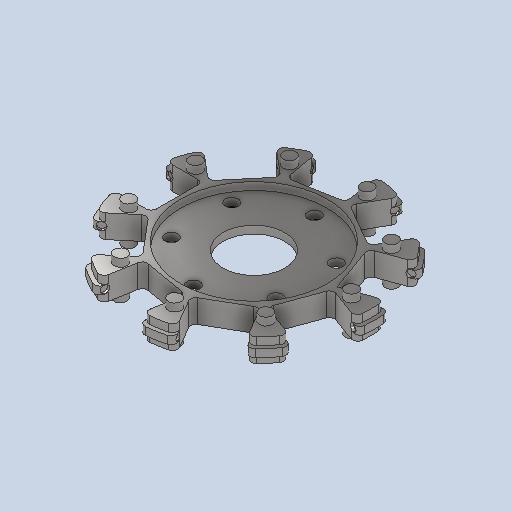
# Autodesk Inventor part: omuni_flame
Saved by Autodesk Inventor 2025.1 (Build 291241000, 241)
## iProperties
Created: 2023-11-21
Part Number: omuni_flame
Material: ステンレス鋼
Document SubType Name: Modeling
Designer: fhbdh
Density: 8 g/cm^3
Appearance: 半つや出し
Author: fhbdh
Autodesk Inventor part; units mm, degrees
ref_plane "YZ Plane" through (0, 0, 0) normal (1, 0, 0) x (0, 1, 0)
ref_plane "XZ Plane" through (0, 0, 0) normal (0, 1, 0) x (-1, 0, 0)
ref_plane "XY Plane" through (0, 0, 0) normal (0, 0, 1) x (1, 0, 0)
sketch "スケッチ1" plane through (0, 0, 0) normal (0, 1, 0) x (-1, 0, 0)
  circle A0 centre (0, 0) radius 12
  circle A1 centre (0, 0) radius 47
  line L0 (45.92385, 10) -> (29.92385, 10)
  line L1 (29.92385, 10) -> (29.92385, -10)
  line L2 (29.92385, -10) -> (45.92385, -10)
  line L3 (0, 0) -> (47, 0) construction
  line L4 (28.751834, 37.179726) -> (16.495123, 26.895124)
  line L5 (16.495123, 26.895124) -> (29.350875, 11.574236)
  line L6 (29.350875, 11.574236) -> (41.607586, 21.858837)
  line L7 (-1.873485, 46.962645) -> (-4.651856, 31.205721)
  line L8 (-4.651856, 31.205721) -> (15.0443, 27.732758)
  line L9 (15.0443, 27.732758) -> (17.82267, 43.489682)
  line L10 (-31.622179, 34.771221) -> (-23.622179, 20.914814)
  line L11 (-23.622179, 20.914814) -> (-6.301671, 30.914814)
  line L12 (-6.301671, 30.914814) -> (-14.301671, 44.771221)
  line L13 (-46.574504, 6.309956) -> (-31.539422, 0.837633)
  line L14 (-31.539422, 0.837633) -> (-24.69902, 19.631486)
  line L15 (-24.69902, 19.631486) -> (-39.734102, 25.103808)
  line L16 (-39.734102, -25.103808) -> (-24.69902, -19.631486)
  line L17 (-24.69902, -19.631486) -> (-31.539422, -0.837633)
  line L18 (-31.539422, -0.837633) -> (-46.574504, -6.309956)
  line L19 (-14.301671, -44.771221) -> (-6.301671, -30.914814)
  line L20 (-6.301671, -30.914814) -> (-23.622179, -20.914814)
  line L21 (-23.622179, -20.914814) -> (-31.622179, -34.771221)
  line L22 (17.82267, -43.489682) -> (15.0443, -27.732758)
  line L23 (15.0443, -27.732758) -> (-4.651856, -31.205721)
  line L24 (-4.651856, -31.205721) -> (-1.873485, -46.962645)
  line L25 (41.607586, -21.858837) -> (29.350875, -11.574236)
  line L26 (29.350875, -11.574236) -> (16.495123, -26.895124)
  line L27 (16.495123, -26.895124) -> (28.751834, -37.179726)
  line L28 (0, 47) -> (0, -47) construction
  circle A2 centre (0, 23.5) radius 2.5
  circle A3 centre (-20.351597, 11.75) radius 2.5
  circle A4 centre (-20.351597, -11.75) radius 2.5
  circle A5 centre (0, -23.5) radius 2.5
  circle A6 centre (20.351597, -11.75) radius 2.5
  circle A7 centre (20.351597, 11.75) radius 2.5
  point P0 (0, 0)
  dimension "d0" = 24
  dimension "d1" = 35
  dimension "d2" = 20
  dimension "d3" = 16
  dimension "d6" = 360
  dimension "d8" = 5
  dimension "d9" = 23.5
  dimension "d12" = 360
  constraints: 58 end point, 8 centre point, 5 point on circle, 2 coincident, 2 horizontal, 2 midpoint, 2 perpendicular, 1 point on line, 1 vertical, 78 other
  measures "d0" diameter of A0
  measures "d1" radial gap between concentric circles of A1 A0
  measures "d2" distance of L0.end L1.end
  measures "d3" distance of L0.start L0.end
  measures "d8" diameter of A2
  measures "d9" distance of point (0, 0) A2.centre
extrude "押し出し1" add sketch "スケッチ1" along normal blind 3 contours L0 L1 L2 A1 L25 L26 L27 L22 L23 L24 L19 L20 L21 L16 L17 L18 L13 L14 L15 L10 L11 L12 L7 L8 L9 L4 L5 L6
fillet "フィレット1" radius 2 36 edges at (6.3017, 1.5, 30.9148) (23.6222, 1.5, 20.9148) (14.3017, 1.5, 44.7712) (31.6222, 1.5, 34.7712) (39.7341, 1.5, 25.1038) (24.699, 1.5, 19.6315) (31.5394, 1.5, 0.8376) (46.5745, 1.5, 6.31) (46.5745, 1.5, -6.31) (31.5394, 1.5, -0.8376) (24.699, 1.5, -19.6315) (23.6222, 1.5, -20.9148) (39.7341, 1.5, -25.1038) (31.6222, 1.5, -34.7712) (6.3017, 1.5, -30.9148) (14.3017, 1.5, -44.7712) (1.8735, 1.5, -46.9626) (4.6519, 1.5, -31.2057) (-15.0443, 1.5, -27.7328) (-16.4951, 1.5, -26.8951) (-17.8227, 1.5, -43.4897) (-28.7518, 1.5, -37.1797) (-29.3509, 1.5, -11.5742) (-41.6076, 1.5, -21.8588) (-45.9239, 1.5, -10) (-29.9239, 1.5, -10) (-29.9239, 1.5, 10) (-45.9239, 1.5, 10) (-41.6076, 1.5, 21.8588) (-29.3509, 1.5, 11.5742) (-16.4951, 1.5, 26.8951) (-28.7518, 1.5, 37.1797) (-17.8227, 1.5, 43.4897) (-15.0443, 1.5, 27.7328) (4.6519, 1.5, 31.2057) (1.8735, 1.5, 46.9626)
sketch "スケッチ2" plane through (0, 3, 0) normal (0, 1, 0) x (1, 0, 0)
  circle A0 centre (0, 0) radius 28.5
  circle A1 centre (0, 0) radius 12
  circle A2 centre (0, 0) radius 45.5
  line L0 (-44.387498, 10) -> (-29.92385, 10)
  line L1 (-29.92385, 10) -> (-29.92385, -10)
  line L2 (-29.92385, -10) -> (-44.387498, -10)
  line L3 (-43.370497, 10) -> (-31.92385, 10)
  line L4 (-29.92385, 8) -> (-29.92385, -8)
  line L5 (-31.92385, -10) -> (-43.370497, -10)
  line L6 (-40.430672, -20.871289) -> (-29.350875, -11.574236)
  line L7 (-29.350875, -11.574236) -> (-16.495123, -26.895124)
  line L8 (-16.495123, -26.895124) -> (-27.57492, -36.192178)
  line L9 (-17.555886, -41.976671) -> (-15.0443, -27.732758)
  line L10 (-15.0443, -27.732758) -> (4.651856, -31.205721)
  line L11 (4.651856, -31.205721) -> (2.140269, -45.449634)
  line L12 (13.533495, -43.440701) -> (6.301671, -30.914814)
  line L13 (6.301671, -30.914814) -> (23.622179, -20.914814)
  line L14 (23.622179, -20.914814) -> (30.854003, -33.440701)
  line L15 (38.290403, -24.578345) -> (24.69902, -19.631486)
  line L16 (24.69902, -19.631486) -> (31.539422, -0.837633)
  line L17 (31.539422, -0.837633) -> (45.130806, -5.784492)
  line L18 (45.130806, 5.784492) -> (31.539422, 0.837633)
  line L19 (31.539422, 0.837633) -> (24.69902, 19.631486)
  line L20 (24.69902, 19.631486) -> (38.290403, 24.578345)
  line L21 (30.854003, 33.440701) -> (23.622179, 20.914814)
  line L22 (23.622179, 20.914814) -> (6.301671, 30.914814)
  line L23 (6.301671, 30.914814) -> (13.533495, 43.440701)
  line L24 (2.140269, 45.449634) -> (4.651856, 31.205721)
  line L25 (4.651856, 31.205721) -> (-15.0443, 27.732758)
  line L26 (-15.0443, 27.732758) -> (-17.555886, 41.976671)
  line L27 (-27.57492, 36.192178) -> (-16.495123, 26.895124)
  line L28 (-16.495123, 26.895124) -> (-29.350875, 11.574236)
  line L29 (-29.350875, 11.574236) -> (-40.430672, 20.871289)
  dimension "d17" = 57
  dimension "d18" = 17
  dimension "d21" = 360
  constraints: 54 end point, 3 collinear, 2 centre point, 2 coincident, 2 perpendicular, 2 point on circle, 1 horizontal, 64 other
  measures "d17" diameter of A0
  measures "d18" radial gap between concentric circles of A2 A0
extrude "押し出し2" add sketch "スケッチ2" along normal blind 3 contours A2 L17 L16 L15 L14 L13 L12 L11 L10 L9 L8 L7 L6 L2 L1 L0 L29 L28 L27 L26 L25 L24 L23 L22 L21 L20 L19 L18
sketch "スケッチ3" plane through (0, 0, 0) normal (0, -1, 0) x (1, 0, 0)
  line L0 (-16.495123, 26.895124) -> (-27.57492, 36.192178)
  arc A0 (-17.555886, 41.976671) -> (-27.57492, 36.192178) centre (0, 0) ccw
  line L1 (-17.555886, 41.976671) -> (-15.0443, 27.732758)
  line L2 (-15.0443, 27.732758) -> (4.651856, 31.205721)
  line L3 (4.651856, 31.205721) -> (2.140269, 45.449634)
  arc A1 (13.533495, 43.440701) -> (2.140269, 45.449634) centre (0, 0) ccw
  line L4 (13.533495, 43.440701) -> (6.301671, 30.914814)
  line L5 (6.301671, 30.914814) -> (23.622179, 20.914814)
  line L6 (23.622179, 20.914814) -> (30.854003, 33.440701)
  arc A2 (38.290403, 24.578345) -> (30.854003, 33.440701) centre (0, 0) ccw
  line L7 (38.290403, 24.578345) -> (24.69902, 19.631486)
  line L8 (24.69902, 19.631486) -> (31.539422, 0.837633)
  line L9 (31.539422, 0.837633) -> (45.130806, 5.784492)
  arc A3 (45.130806, -5.784492) -> (45.130806, 5.784492) centre (0, 0) ccw
  line L10 (45.130806, -5.784492) -> (31.539422, -0.837633)
  line L11 (31.539422, -0.837633) -> (24.69902, -19.631486)
  line L12 (24.69902, -19.631486) -> (38.290403, -24.578345)
  arc A4 (30.854003, -33.440701) -> (38.290403, -24.578345) centre (0, 0) ccw
  line L13 (30.854003, -33.440701) -> (23.622179, -20.914814)
  line L14 (23.622179, -20.914814) -> (6.301671, -30.914814)
  line L15 (6.301671, -30.914814) -> (13.533495, -43.440701)
  arc A5 (2.140269, -45.449634) -> (13.533495, -43.440701) centre (0, 0) ccw
  line L16 (2.140269, -45.449634) -> (4.651856, -31.205721)
  line L17 (4.651856, -31.205721) -> (-15.0443, -27.732758)
  line L18 (-15.0443, -27.732758) -> (-17.555886, -41.976671)
  arc A6 (-27.57492, -36.192178) -> (-17.555886, -41.976671) centre (0, 0) ccw
  line L19 (-27.57492, -36.192178) -> (-16.495123, -26.895124)
  line L20 (-16.495123, -26.895124) -> (-29.350875, -11.574236)
  line L21 (-29.350875, -11.574236) -> (-40.430672, -20.871289)
  arc A7 (-44.387498, -10) -> (-40.430672, -20.871289) centre (0, 0) ccw
  line L22 (-44.387498, -10) -> (-29.92385, -10)
  line L23 (-29.92385, -10) -> (-29.92385, 10)
  line L24 (-29.92385, 10) -> (-44.387498, 10)
  arc A8 (-40.430672, 20.871289) -> (-44.387498, 10) centre (0, 0) ccw
  line L25 (-40.430672, 20.871289) -> (-29.350875, 11.574236)
  line L26 (-29.350875, 11.574236) -> (-16.495123, 26.895124)
  circle A9 centre (0, 0) radius 28.5
extrude "押し出し3" add sketch "スケッチ3" along normal blind 3
fillet "フィレット2" radius 2 50 edges at (2.1403, -1.5, 45.4496) (2.1403, 4.5, 45.4496) (4.6519, -1.5, 31.2057) (4.6519, 4.5, 31.2057) (13.5335, 4.5, 43.4407) (13.5335, -1.5, 43.4407) (6.3017, -1.5, 30.9148) (6.3017, 4.5, 30.9148) (23.6222, 4.5, 20.9148) (23.6222, -1.5, 20.9148) (30.854, -1.5, 33.4407) (30.854, 4.5, 33.4407) (38.2904, -1.5, 24.5783) (38.2904, 4.5, 24.5783) (24.699, -1.5, 19.6315) (24.699, 4.5, 19.6315) (31.5394, -1.5, 0.8376) (31.5394, 4.5, 0.8376) (45.1308, 4.5, 5.7845) (45.1308, -1.5, 5.7845) (45.1308, 4.5, -5.7845) (45.1308, -1.5, -5.7845) (38.2904, 4.5, -24.5783) (38.2904, -1.5, -24.5783) (24.699, -1.5, -19.6315) (24.699, 4.5, -19.6315) (23.6222, 4.5, -20.9148) (23.6222, -1.5, -20.9148) (30.854, -1.5, -33.4407) (30.854, 4.5, -33.4407) (6.3017, 4.5, -30.9148) (6.3017, -1.5, -30.9148) (13.5335, -1.5, -43.4407) (13.5335, 4.5, -43.4407) (2.1403, -1.5, -45.4496) (2.1403, 4.5, -45.4496) (4.6519, -1.5, -31.2057) (4.6519, 4.5, -31.2057) (-17.5559, -1.5, -41.9767) (-17.5559, 4.5, -41.9767) (-15.0443, -1.5, -27.7328) (-15.0443, 4.5, -27.7328) (-27.5749, -1.5, -36.1922) (-27.5749, 4.5, -36.1922) (-16.4951, -1.5, -26.8951) (-16.4951, 4.5, -26.8951) (-29.3509, -1.5, -11.5742) (-29.3509, 4.5, -11.5742) (-40.4307, -1.5, -20.8713) (-40.4307, 4.5, -20.8713)
fillet "フィレット3" radius 2 20 edges at (-44.3875, -1.5, -10) (-44.3875, 4.5, -10) (-29.9239, -1.5, -10) (-29.9239, 4.5, -10) (-44.3875, -1.5, 10) (-44.3875, 4.5, 10) (-29.9239, -1.5, 10) (-29.9239, 4.5, 10) (-40.4307, -1.5, 20.8713) (-40.4307, 4.5, 20.8713) (-29.3509, -1.5, 11.5742) (-29.3509, 4.5, 11.5742) (-16.4951, -1.5, 26.8951) (-16.4951, 4.5, 26.8951) (-27.5749, 4.5, 36.1922) (-27.5749, -1.5, 36.1922) (-17.5559, -1.5, 41.9767) (-17.5559, 4.5, 41.9767) (-15.0443, 4.5, 27.7328) (-15.0443, -1.5, 27.7328)
sketch "スケッチ4" plane through (2.31687, 0, 44.448083) normal (-0.9848078, 0, -0.1736482) x (-0.1736482, 0, 0.9848078)
  circle A0 centre (-0.446647, 1.5) radius 1.5
  line L0 (1.927578, 0) -> (1.927578, 3)
  point P0 (-43.370497, 0)
  point P1 (-13.446647, 6)
  point P2 (1.927578, 1.5)
  dimension "d29" = 3
  dimension "d30" = 13
  dimension "d31" = 0
  constraints: 1 centre point, 1 midpoint
  measures "d29" diameter of A0
  measures "d30" horizontal distance of A0.centre point (-13.447, 6)
  measures "d31" vertical distance of point (1.928, 1.5) A0.centre
extrude "押し出し4" cut sketch "スケッチ4" against normal blind 1
pattern_circular "円形状パターン1" count 9 over 360 about axis through (0, 0, 0) along (0, 1, 0) of "押し出し4"
sketch "スケッチ5" plane through (-17.379285, 0, 40.97512) normal (0.9848078, 0, 0.1736482) x (0.1736482, 0, -0.9848078)
  circle A0 centre (0.446647, 1.5) radius 1.5
  line L0 (0, 0) -> (0, 3)
  point P0 (43.370497, 0)
  point P1 (13.446647, 6)
  point P2 (0, 1.5)
  dimension "d37" = 3
  dimension "d38" = 13
  dimension "d39" = 0
  constraints: 1 centre point, 1 midpoint
  measures "d37" diameter of A0
  measures "d38" horizontal distance of point (13.447, 6) A0.centre
  measures "d39" vertical distance of point (0, 1.5) A0.centre
extrude "押し出し5" cut sketch "スケッチ5" against normal blind 1
pattern_circular "円形状パターン2" count 9 over 360 about axis through (0, 0, 0) along (0, 1, 0) of "押し出し5"
sketch "スケッチ6" plane through (0, 6, 0) normal (0, 1, 0) x (1, 0, 0)
  circle A0 centre (38, 0) radius 2.5
  circle A1 centre (0, 0) radius 28.5
  line L0 (28.5, 0) -> (-28.5, 0) construction
  circle A2 centre (29.109689, 24.425929) radius 2.5
  circle A3 centre (6.598631, 37.422695) radius 2.5
  circle A4 centre (-19, 32.908965) radius 2.5
  circle A5 centre (-35.70832, 12.996765) radius 2.5
  circle A6 centre (-35.70832, -12.996765) radius 2.5
  circle A7 centre (-19, -32.908965) radius 2.5
  circle A8 centre (6.598631, -37.422695) radius 2.5
  circle A9 centre (29.109689, -24.425929) radius 2.5
  dimension "d45" = 5
  dimension "d46" = 38
  dimension "d49" = 360
  constraints: 9 centre point, 2 end point, 2 midpoint, 2 point on circle, 1 horizontal, 1 point on line, 19 other
  measures "d45" diameter of A0
  measures "d46" distance of point (0, 0) A0.centre
extrude "押し出し6" add sketch "スケッチ6" along normal blind 3 contours A0 | A2 | A3 | A4 | A5 | A6 | A7 | A8 | A9
sketch "スケッチ7" plane through (0, -3, 0) normal (0, -1, 0) x (1, 0, 0)
  circle A0 centre (38, 0) radius 2.5
  circle A1 centre (6.598631, 37.422695) radius 2.5
  circle A2 centre (-19, 32.908965) radius 2.5
  circle A3 centre (-35.70832, 12.996765) radius 2.5
  circle A4 centre (-35.70832, -12.996765) radius 2.5
  circle A5 centre (-19, -32.908965) radius 2.5
  circle A6 centre (6.598631, -37.422695) radius 2.5
  circle A7 centre (29.109689, -24.425929) radius 2.5
  circle A8 centre (29.109689, 24.425929) radius 2.5
  point P0 (0, 0)
extrude "押し出し7" add sketch "スケッチ7" along normal blind 3
